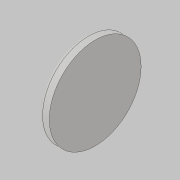
# Autodesk Inventor part: Connector_box_collar-None
Saved by Autodesk Inventor 2019.3 (Build 233278000, 278)
## iProperties
Created: 2019-02-06
Part Number: Connector_box_collar-None
Material: Generic
Document SubType Name: Modeling
Designer: Varga Daniel
Density: 1 g/cm^3
Appearance: Default
Author: Varga Daniel
Autodesk Inventor part; units mm, degrees
ref_plane "YZ Plane" through (0, 0, 0) normal (1, 0, 0) x (0, 1, 0)
ref_plane "XZ Plane" through (0, 0, 0) normal (0, 1, 0) x (-1, 0, 0)
derived "Connector_pin_base.ipt"
sketch "Pin_base_sketch" plane through (0, 0, 0) normal (0, 0, 1) x (1, 0, 0)
  line L0 (0, 0) -> (23.0918, 0) construction
  line L1 (0, 0) -> (0, 6.22) construction
  line L2 (0, 3.75) -> (0.55, 3.75)
  line L3 (0.85, 3.45) -> (0.85, 2.4375)
  line L4 (0.85, 2.4375) -> (10.1, 2.4375)
  line L5 (10.1, 2.4375) -> (10.1, 0)
  line L6 (0, 0) -> (0, 3.75)
  line L7 (0, 0) -> (10.1, 0)
  line L8 (9.35, 2.4375) -> (9.35, 2.625)
  line L9 (10.1, 2.4375) -> (10.1, 2.4399)
  arc A0 (10.1, 2.4399) -> (9.9105, 2.7318) centre (9.7805, 2.4399) ccw
  arc A1 (9.9105, 2.7318) -> (9.35, 2.625) centre (9.7071, 2.275) ccw
  line L10 (9.9105, 2.7318) -> (9.9105, -0.0075) construction
  line L11 (8.9584, 2.775) -> (10.3858, 2.775) construction
  arc A2 (0.85, 3.45) -> (0.55, 3.75) centre (0.55, 3.45) ccw
  line L12 (0.85, 2.4375) -> (0.85, 0)
  line L13 (-0.85, 2.4375) -> (-0.85, 0)
  line L14 (-0.85, 3.45) -> (-0.85, 2.4375)
  arc A3 (-0.55, 3.75) -> (-0.85, 3.45) centre (-0.55, 3.45) ccw
  line L15 (0, 3.75) -> (-0.55, 3.75)
  line L16 (0, 0) -> (-23.0918, 0) construction
  line L17 (0, 0) -> (-10.1, 0)
  line L18 (-0.85, 2.4375) -> (-10.1, 2.4375)
  line L19 (-9.35, 2.4375) -> (-9.35, 2.625)
  arc A4 (-9.35, 2.625) -> (-9.9105, 2.7318) centre (-9.7071, 2.275) ccw
  arc A5 (-9.9105, 2.7318) -> (-10.1, 2.4399) centre (-9.7805, 2.4399) ccw
  line L20 (-10.1, 2.4375) -> (-10.1, 2.4399)
  line L21 (-8.9584, 2.775) -> (-10.3858, 2.775) construction
  line L22 (-9.9105, 2.7318) -> (-9.9105, -0.0075) construction
  line L23 (-10.1, 2.4375) -> (-10.1, 0)
  line L24 (9.725, 3.2563) -> (9.725, -1.1868) construction
  dimension "d2" = 0.85
  dimension "d3" = 0.3
  dimension "d7" = 7.5
  measures "d2" distance between parallel lines of L3 L1
  measures "d3" radius of A2
  measures "d7" diameter of L2 L0
derived "beam_single_end_part.ipt"
sketch "Sketch3" plane through (0, 0, 0) normal (0, 1, 0) x (-1, 0, 0)
  circle A0 centre (5, 5) radius 2.5 construction
  circle A1 centre (5, 5) radius 3.5 construction
  arc A2 (2.5, 5) -> (5, 7.5) centre (5, 5) ccw
  arc A3 (4.5, 1.5359) -> (5.5, 1.5359) centre (5, 5) ccw
  line L0 (0.3508, 5) -> (13.598, 5) construction
  line L1 (5, 13.9543) -> (5, -1.7484) construction
  line L2 (5, 10) -> (0, 10)
  line L3 (0, 10) -> (0, 9)
  line L4 (0, 9) -> (0, 9)
  line L5 (0, 1) -> (0, 0)
  line L6 (0, 0) -> (5, 0)
  line L7 (0, 0) -> (0, 1)
  line L8 (1.5359, 5.5) -> (0, 5.5)
  line L9 (0, 5.5) -> (0, 4.5)
  line L10 (0, 4.5) -> (1.5359, 4.5)
  line L11 (0, 9) -> (4.5, 9)
  line L12 (0, 9) -> (0, 10)
  line L13 (5, 9) -> (5, 9)
  line L14 (5, 1) -> (4.5, 1)
  arc A4 (5, 1) -> (5.5, 1.0314) centre (5, 5) ccw
  line L15 (4.5, 9) -> (4.5, 8.4641)
  line L16 (5.5, 8.9686) -> (5.5, 8.4641)
  line L17 (5.5, 1.0314) -> (5.5, 1.5359)
  line L18 (4.5, 1.5359) -> (4.5, 1)
  line L19 (8.4641, 5.5) -> (8.9686, 5.5)
  line L20 (8.4641, 4.5) -> (8.9686, 4.5)
  line L21 (0, 1) -> (0, 4.5)
  line L22 (0, 4.5) -> (0, 5.5)
  line L23 (0, 5.5) -> (0, 9)
  line L24 (4.5, 9) -> (5, 9)
  arc A5 (8.9686, 5.5) -> (5.5, 8.9686) centre (5, 5) ccw
  arc A6 (8.9686, 4.5) -> (8.9686, 5.5) centre (5, 5) ccw
  arc A7 (1.5359, 4.5) -> (4.5, 1.5359) centre (5, 5) ccw
  arc A8 (1.5359, 5.5) -> (1.5359, 4.5) centre (5, 5) ccw
  line L25 (4.5, 1) -> (0, 1)
  line L26 (0, 9) -> (4.5, 9)
  line L27 (4.5, 9) -> (5, 9)
  circle A9 centre (5, 5) radius 2.5 construction
  arc A10 (10, 5) -> (5, 10) centre (5, 5) ccw
  arc A11 (5, 0) -> (10, 5) centre (5, 5) ccw
  arc A12 (5.5, 8.9686) -> (5, 9) centre (5, 5) ccw
  arc A13 (8.4641, 5.5) -> (5.5, 8.4641) centre (5, 5) ccw
  arc A14 (5.5, 8.4641) -> (4.5, 8.4641) centre (5, 5) ccw
  arc A15 (5.5, 1.0314) -> (8.9686, 4.5) centre (5, 5) ccw
  arc A16 (8.4641, 4.5) -> (8.4641, 5.5) centre (5, 5) ccw
  arc A17 (4.5, 8.4641) -> (1.5359, 5.5) centre (5, 5) ccw
  arc A18 (5.5, 1.5359) -> (8.4641, 4.5) centre (5, 5) ccw
  arc A19 (5, 7.5) -> (2.5, 5) centre (5, 5) ccw
  point P0 (0, 0)
ref_plane "Work Plane4" through (-10, 0, 5) normal (-1, 0, 0) x (0, -1, 0)
sketch "Sketch4" plane through (-10, 0, 5) normal (-1, 0, 0) x (0, -1, 0)
  line L0 (0, 0) -> (0, -5) projected
  line L1 (0, 5) -> (0, 0) projected
  arc A0 (0, -3.75) -> (3.75, 0) centre (0, 0) ccw
  line L2 (3.75, 0) -> (-3.75, 0)
  arc A1 (-3.75, 0) -> (0, -3.75) centre (0, 0) ccw
  arc A2 (3.75, 0) -> (0, 3.75) centre (0, 0) ccw
  arc A3 (0, 3.75) -> (-3.75, 0) centre (0, 0) ccw
  dimension "d15" = 7.5
  constraints: 8 point on circle, 4 centre point, 2 end point, 2 point on line, 1 coincident, 1 horizontal, 1 midpoint, 1 perpendicular
  measures "d15" diameter of A0
extrude "Extrusion4" add sketch "Sketch4" along normal blind 0.85
fillet "Fillet2" radius 0.3 4 edges at (-10.85, 2.6517, 2.3483) (-10.85, 2.6517, 7.6517) (-10.85, -2.6517, 2.3483) (-10.85, -2.6517, 7.6517)
extrude "Extrusion5" [suppressed]
extrude "Extrusion6" [suppressed]
extrude "Extrusion7" [suppressed]
equation "\"d15\" = d7"
equation "\"d16\" = d2"
equation "\"d18\" = d3"
body "Solid3"
